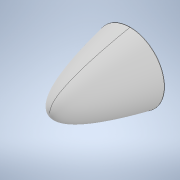
# Autodesk Inventor part: Spitze
Saved by Autodesk Inventor 2020 (Build 240168000, 168)
## iProperties
Created: 2022-01-25
Part Number: Spitze
Material: Generisch
Document SubType Name: Modeling
Designer: sp
Density: 1 g/cm^3
Appearance: Vorgabe
Author: sp
Autodesk Inventor part; units mm, degrees
ref_plane "YZ Plane" through (0, 0, 0) normal (1, 0, 0) x (0, 1, 0)
ref_plane "XZ Plane" through (0, 0, 0) normal (0, 1, 0) x (-1, 0, 0)
ref_plane "XY Plane" through (0, 0, 0) normal (0, 0, 1) x (1, 0, 0)
sketch "Skizze1" plane through (0, 0, 0) normal (1, 0, 0) x (0, 1, 0)
  line L0 (0, 2094.1927) -> (0, -1699.1575) construction
  line L1 (933.6484, 0) -> (-899.755, 0) construction
  spline S0 degree 2 poles (33, 0) (0, 160) (-33, 0) knots 0 0 0 1 1 1
  line L2 (0, 90.8614) -> (0, 0)
  line L3 (0, 0) -> (44.134, 0)
  line L4 (34.9588, 0.404) -> (34.9588, 0)
  line L5 (-34.9588, 0.404) -> (-34.9588, 0)
  spline S1 degree 5 poles (34.9588, 0.404) (34.0777, 4.6757) (33.1686, 8.9415) (32.2277, 13.2006) (30.4147, 21.0886) (28.4525, 28.9408) (27.5115, 32.5523) (25.7082, 39.1559) (23.7297, 45.7089) (22.7876, 48.6763) (20.9941, 54.0116) (18.9891, 59.2707) (18.043, 61.6011) (16.2512, 65.7026) (14.1966, 69.6778) (13.2348, 71.3856) (11.4014, 74.3287) (9.2284, 77.0292) (8.2102, 78.1377) (6.1495, 80.0074) (3.7107, 81.3274) (2.5127, 81.776) (0, 82.224) (-2.5127, 81.776) (-3.7107, 81.3274) (-6.1495, 80.0074) (-8.2102, 78.1377) (-9.2284, 77.0292) (-11.4014, 74.3287) (-13.2348, 71.3856) (-14.1966, 69.6778) (-16.2512, 65.7026) (-18.043, 61.6011) (-18.9891, 59.2707) (-20.9941, 54.0116) (-22.7876, 48.6763) (-23.7297, 45.7089) (-25.7082, 39.1559) (-27.5115, 32.5523) (-28.4525, 28.9408) (-30.4147, 21.0886) (-32.2277, 13.2006) (-33.1686, 8.9415) (-34.0777, 4.6757) (-34.9588, 0.404) knots 0 0 0 0 0 0 0.118283 0.118283 0.118283 0.219486 0.219486 0.219486 0.303907 0.303907 0.303907 0.372097 0.372097 0.372097 0.425208 0.425208 0.425208 0.46594 0.46594 0.46594 0.5 0.5 0.5 0.53406 0.53406 0.53406 0.574792 0.574792 0.574792 0.627903 0.627903 0.627903 0.696093 0.696093 0.696093 0.780514 0.780514 0.780514 0.881717 0.881717 0.881717 1 1 1 1 1 1
  point P0 (0, 80)
  point P1 (0, 82)
  point P2 (0, 80)
  point P3 (33, 0)
  dimension "d5" = 2
  dimension "d2" = 80
  dimension "d3" = 33
  dimension "d4" = 33
  constraints: 12 end point, 9 point on line, 3 perpendicular, 1 horizontal, 1 vertical, 6 other
  measures "d2" distance of point (0, 80) L2.end
  measures "d3" distance of L2.end point (33, 0)
  measures "d4" distance of point (-33, 0) L2.end
revolve "Umdrehung1" add sketch "Skizze1" angle 360 about axis through (0, 0, 2094.1927) along (0, 0, -1) contours S0 L2 S1 L4 L3
